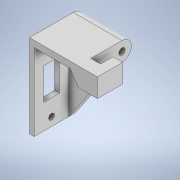
# Autodesk Inventor part: Pi3B_spacer_R_switch
Saved by Autodesk Inventor 2022 (Build 260153000, 153)
## iProperties
Created: 2023-01-27
Part Number: Pi3B_spacer_R_switch
Material: Generic
Document SubType Name: Modeling
Designer: scott
Density: 1 g/cm^3
Appearance: Default
Author: scott
Autodesk Inventor part; units mm, degrees
ref_plane "YZ Plane" through (0, 0, 0) normal (1, 0, 0) x (0, 1, 0)
ref_plane "XZ Plane" through (0, 0, 0) normal (0, 1, 0) x (-1, 0, 0)
ref_plane "XY Plane" through (0, 0, 0) normal (0, 0, 1) x (1, 0, 0)
sketch "Sketch1" plane through (0, 0, 0) normal (0, 1, 0) x (-1, 0, 0)
  line L0 (0, 0) -> (21.6, 0)
  line L1 (21.6, 0) -> (21.6, 17)
  line L2 (21.6, 17) -> (0, 17)
  line L3 (0, 17) -> (0, 0)
  line L4 (6.1, 13) -> (3, 13)
  line L5 (3, 13) -> (3, 0)
  line L6 (3, 0) -> (6.1, 0)
  line L7 (6.1, 0) -> (6.1, 13)
  line L8 (21.6, 17) -> (9.1, 17)
  line L9 (9.1, 17) -> (9.1, 0)
  line L10 (9.1, 0) -> (21.6, 0)
  line L11 (21.6, 0) -> (21.6, 17)
  line L12 (9.1, 17) -> (21.6, 6.2)
  point P0 (21.6, 6.2)
  point P1 (9.1, 17)
  dimension "d1" = 17
  dimension "d2" = 3.1
  dimension "d3" = 3
  dimension "d4" = 3
  dimension "d5" = 6.2
  dimension "d17" = 13
  dimension "d18" = 12.5
  constraints: 26 end point, 6 parallel, 3 horizontal, 3 perpendicular, 3 point on line
  measures "d1" distance of L1.end L0.end
  measures "d2" distance between parallel lines of L5 L7
  measures "d3" distance between parallel lines of L3 L5
  measures "d4" distance between parallel lines of L7 L9
  measures "d5" distance from line of L0 L12.end
  measures "d17" distance between parallel lines of L0 L4
  measures "d18" distance between parallel lines of L9 L1
extrude "Extrusion1" add sketch "Sketch1" along normal blind 6 contours L3 L2 L9 L0 L7 L4 L5 | L12 L1 L0 L9
sketch "Sketch2" plane through (-21.6, 0, 0) normal (-1, 0, 0) x (0, 0, 1)
  circle A0 centre (3.1, 3) radius 3
  line L0 (0, 0) -> (13, 0) projected
  line L1 (0, 0) -> (0, 6) projected
  line L2 (17, 6) -> (0, 6) projected
  line L3 (0, 0) -> (6.2302, 0)
  line L4 (6.2302, 0) -> (6.2302, 6)
  line L5 (6.2302, 6) -> (0, 6)
  line L6 (0, 6) -> (0, 0)
  circle A1 centre (3.1, 3) radius 1
  point P0 (3.1, 6)
  point P1 (3.1, 0)
  dimension "d8" = 3.1
  dimension "d9" = 2
  constraints: 8 end point, 2 centre point, 2 parallel, 1 coincident, 1 horizontal, 1 perpendicular, 1 point on line, 1 tangent
  measures "d8" distance from line of L1 A0.centre
  measures "d9" diameter of A1
extrude "Extrusion2" cut sketch "Sketch2" against normal up to surface (18.6 mm away) contours A0 L0 L1 L2 | A1
sketch "Sketch3" plane through (0, 6, 0) normal (0, 1, 0) x (1, 0, 0)
  line L0 (-3, 0) -> (-3, -13) projected
  line L1 (0, 0) -> (-3, 0) projected
  line L2 (-3, -9) -> (0, -9)
  line L3 (0, -9) -> (0, 0)
  line L4 (0, 0) -> (-3, 0)
  line L5 (-3, 0) -> (-3, -9)
  line L6 (-3, -13) -> (-6.1, -13) projected
  line L7 (-9.1, -17) -> (0, -17) projected
  dimension "d13" = 8
  constraints: 8 end point, 2 parallel, 1 horizontal, 1 perpendicular, 1 point on line
  measures "d13" distance between parallel lines of L7 L2
extrude "Extrusion3" cut sketch "Sketch3" against normal blind 10
sketch "Sketch4" plane through (0, 0, 0) normal (0, -1, 0) x (1, 0, 0)
  line L0 (-21.6, 6.2) -> (-9.1, 17) projected
  line L1 (-9.1, 17) -> (-20.1, 17)
  line L2 (-20.1, 17) -> (-20.1, 7.496)
  line L3 (-20.1, 7.496) -> (-9.1, 7.496)
  line L4 (-9.1, 7.496) -> (-9.1, 17)
  line L5 (-6.1, 13) -> (-6.1, 3.1) projected
  point P0 (0, 0)
  dimension "d19" = 14
  constraints: 8 end point, 2 parallel, 1 horizontal, 1 perpendicular, 1 point on line
  measures "d19" distance between parallel lines of L5 L2
extrude "Extrusion4" cut sketch "Sketch4" against normal blind 4 contours L0 L4 L3
sketch "Sketch5" plane through (0, 0, 0) normal (0, -1, 0) x (1, 0, 0)
  line L0 (-9.1, 17) -> (-9.1, 7.496) projected
  line L1 (-9.1, 17) -> (-8.6, 17)
  line L2 (-8.6, 17) -> (-8.6, 7.496)
  line L3 (-8.6, 7.496) -> (-9.1, 7.496)
  line L4 (-9.1, 7.496) -> (-9.1, 17)
  line L5 (-6.1, 13) -> (-6.1, 3.1) projected
  point P0 (0, 0)
  dimension "d22" = 2.5
  constraints: 8 end point, 2 parallel, 1 horizontal, 1 perpendicular
  measures "d22" distance between parallel lines of L2 L5
extrude "Extrusion5" cut sketch "Sketch5" against normal up to surface (4 mm away)
sketch "Sketch7" plane through (0, 4, 0) normal (0, -1, 0) x (1, 0, 0)
  line L0 (-8.6, 7.496) -> (-8.6, 17) projected
  line L1 (-8.6, 17) -> (-20.1, 17)
  line L2 (-20.1, 17) -> (-20.1, 6)
  line L3 (-20.1, 6) -> (-8.6, 6)
  line L4 (-8.6, 6) -> (-8.6, 17)
  point P0 (0, 0)
  dimension "d25" = 11.5
  dimension "d26" = 11
  constraints: 8 end point, 2 parallel, 1 horizontal, 1 perpendicular
  measures "d25" distance of L3.end L2.end
  measures "d26" distance of L2.end L1.end
extrude "Extrusion6" cut sketch "Sketch7" along normal blind 10
sketch "Sketch8" plane through (0, 4, 0) normal (0, -1, 0) x (1, 0, 0)
  line L0 (-20.1, 7.496) -> (-20.1, 6) projected
  line L1 (-8.6, 6) -> (-8.6, 17) projected
  line L2 (-20.1, 6) -> (-8.6, 6)
  line L3 (-8.6, 6) -> (-8.6, 17)
  line L4 (-8.6, 17) -> (-20.1, 17)
  line L5 (-20.1, 17) -> (-20.1, 6)
  point P0 (0, 0)
  constraints: 8 end point, 2 parallel, 1 horizontal, 1 perpendicular
extrude "Extrusion7" add sketch "Sketch8" against normal up to surface (2 mm away)
sketch "Sketch9" plane through (0, 6, 0) normal (0, 1, 0) x (1, 0, 0)
  line L0 (-20.1, -17) -> (-20.1, -7.496) projected
  line L1 (-21.6, -3.1) -> (-21.6, -6.2) projected
  line L2 (-20.1, -17) -> (-21.6, -17)
  line L3 (-21.6, -17) -> (-21.6, -6)
  line L4 (-21.6, -6) -> (-20.1, -6)
  line L5 (-20.1, -6) -> (-20.1, -17)
  point P0 (0, 0)
  dimension "d31" = 11
  constraints: 8 end point, 2 parallel, 1 horizontal, 1 perpendicular, 1 point on line
  measures "d31" distance of L2.end L3.end
extrude "Extrusion8" add sketch "Sketch9" against normal blind 26.5
sketch "Sketch11" plane through (-20.1, 0, 6) normal (0, 0, -1) x (-1, 0, 0)
  line L0 (0, -20.5) -> (1.5, -20.5) projected
  line L1 (1.5, -20.5) -> (-13.9653, -20.5)
  line L2 (-13.9653, -20.5) -> (-13.9653, 0)
  line L3 (-13.9653, 0) -> (1.5, 0)
  line L4 (1.5, 0) -> (1.5, -20.5)
  line L5 (-13.9653, 0) -> (0, -20.5)
  point P0 (-20.1, 0)
  constraints: 10 end point, 2 parallel, 1 horizontal, 1 perpendicular
extrude "Extrusion9" add sketch "Sketch11" along normal blind 2 contours L5 L3 L4 L0
sketch "Sketch13" plane through (-20.1, 4, 17) normal (1, 0, 0) x (0, 0, -1)
  circle A0 centre (5.5, -2.75) radius 0.9
  circle A1 centre (5.5, -21.75) radius 0.9
  line L0 (11, -24.5) -> (0, -24.5) projected
  line L1 (0, 0) -> (11, 0) projected
  line L2 (8, -6.5185) -> (3, -6.5185)
  line L3 (3, -6.5185) -> (3, -16.5185)
  line L4 (3, -16.5185) -> (8, -16.5185)
  line L5 (8, -16.5185) -> (8, -6.5185)
  line L6 (0, 0) -> (0, -24.5) projected
  point P0 (17, -4)
  dimension "d36" = 2.75
  dimension "d37" = 2.75
  dimension "d38" = 1.8
  dimension "d39" = 1.8
  dimension "d40" = 10
  dimension "d41" = 5
  dimension "d42" = 3
  dimension "d43" = 5.5
  dimension "d44" = 5.5
  constraints: 8 end point, 2 centre point, 2 parallel, 1 horizontal, 1 perpendicular
  measures "d36" distance from line of L0 A1.centre
  measures "d37" distance from line of L1 A0.centre
  measures "d38" diameter of A0
  measures "d39" diameter of A1
  measures "d40" distance of L4.end L2.start
  measures "d41" distance of L3.end L4.end
  measures "d42" distance between parallel lines of L6 L3
  measures "d43" distance from line of L6 A1.centre
  measures "d44" distance from line of L6 A0.centre
extrude "Extrusion10" cut sketch "Sketch13" against normal blind 2
chamfer "Chamfer1" distance 2.5 distance2 4 1 edges at (-8.6, 0, 11.5) measured on face at (-8.1, 0, 11.5)
body "Solid1"
